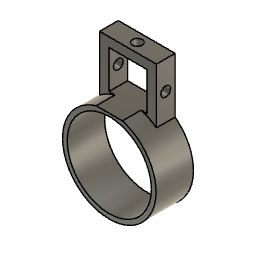
BG브라켓-B (Autodesk Fusion 360 design; units mm, degrees)
Autodesk Fusion 360 part; units mm, degrees
sketch "스케치1" plane through (0, 0, 0) normal (0, 1, 0) x (1, 0, 0)
  circle A0 centre (0, 0) radius 22.5
  line L0 (0, 0) -> (0, -24)
  line L1 (0, -24) -> (15.2, -24)
  line L2 (15.2, -24) -> (-15.2, -24)
  line L3 (-15.2, -24) -> (-15.2, -49.4)
  line L4 (-15.2, -49.4) -> (15.2, -49.4)
  line L5 (15.2, -49.4) -> (15.2, -24)
  circle A1 centre (0, 0) radius 25
  line L6 (-15.2, -24) -> (-15.2, -18.5)
  line L7 (15.2, -24) -> (15.2, -18.5685)
  line L8 (0, -36.7) -> (0, -34.2)
  line L9 (10.2, -44.4) -> (-10.2, -44.4)
  line L10 (-10.2, -44.4) -> (-10.2, -24)
  line L11 (-10.2, -24) -> (10.2, -24)
  line L12 (10.2, -24) -> (10.2, -44.4)
  line L13 (10.2, -44.4) -> (-10.2, -24) construction
  line L14 (-10.2, -44.4) -> (10.2, -24) construction
  point P0 (0, -36.7)
  point P1 (0, -34.2)
  dimension "d1" = 45
  dimension "d2" = 24
  dimension "d3" = 15.2
  dimension "d4" = 30.4
  dimension "d5" = 25.4
  dimension "d8" = 50
  dimension "d13" = 2.5
  dimension "d14" = 20.4
  dimension "d15" = 20.4
  constraint coincident A0.centre L0.start
  constraint vertical L0
  constraint perpendicular L0 L1
  constraint horizontal L2
  constraint vertical L3
  constraint horizontal L4
  constraint vertical L5
  constraint concentric A0 A1
  constraint perpendicular L2 L6
  constraint vertical L7
  constraint coincident P0 L8.start
  constraint vertical L8
  constraint horizontal L9
  constraint perpendicular L9 L10
  constraint parallel L9 L11
  constraint parallel L10 L12
  constraint coincident L13 P1
  constraint coincident L14 P1
  constraint coincident P1 L8.end
  measures "d1" diameter of A0
  measures "d2" distance of A0.centre L0.end
  measures "d3" distance of L0.end L1.end
  measures "d4" distance of L1.end L2.end
  measures "d5" distance of L1.end L4.end
  measures "d8" diameter of A1
  measures "d13" distance of P0 P1
  measures "d14" distance of L10.end L11.end
  measures "d15" distance of L9.end L10.end
extrude "돌출1" add sketch "스케치1" along normal blind 10 contours L1 L2 A1 L7 L11 | L1 L2 L3 L4 L5 L9 L10 L12 | L1 L2 A1 L11 | L2 A1 L6 L11 picked at (-16.0726, -17.9881)
extrude "돌출2" add sketch "스케치1" against normal blind 10 contours L1 L2 A1 L11 picked at (-16.0726, -17.9881)
sketch "스케치2" plane through (0, 0, 49.4) normal (0, 0, 1) x (-1, 0, 0)
  line L0 (15.2, 0) -> (-15.2, 0)
  line L1 (-15.2, 0) -> (-15.2, -10)
  line L2 (-15.2, -10) -> (15.2, -10)
  line L3 (15.2, -10) -> (15.2, 0)
  circle A0 centre (0, -5) radius 2.6
  dimension "d18" = 5.2
  measures "d18" diameter of A0
extrude "돌출3" cut sketch "스케치2" against normal blind 11 contours A0
sketch "스케치3" plane through (-10.2, 0, 0) normal (1, 0, 0) x (0, 1, 0)
  line L0 (0, 44.4) -> (0, 24)
  line L1 (0, 24) -> (10, 24)
  line L2 (10, 24) -> (10, 44.4)
  line L3 (10, 44.4) -> (0, 44.4)
  circle A0 centre (5, 34.2) radius 2.6
  dimension "d21" = 5.2
  measures "d21" diameter of A0
extrude "돌출4" cut sketch "스케치3" along normal blind 33 contours A0
extrude "돌출5" cut sketch "스케치3" against normal blind 17 contours A0
